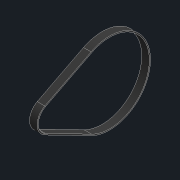
# Autodesk Inventor part: belt_1
Saved by Autodesk Inventor 2022 (Build 260153000, 153)
## iProperties
Created: 2021-07-18
Part Number: belt_1
Material: ゴム
Document SubType Name: Modeling
Designer: yuta0
Density: 0.93 g/cm^3
Appearance: ゴム - 黒
Mass: 8.55769 g
Surface Area: 248.449 cm^2
Volume: 9.20182 cm^3
購入先: ミスミ
在庫数: 0.0
Author: yuta0
Autodesk Inventor part; units mm, degrees
ref_plane "YZ Plane" through (0, 0, 0) normal (1, 0, 0) x (0, 1, 0)
ref_plane "XZ Plane" through (0, 0, 0) normal (0, 1, 0) x (-1, 0, 0)
ref_plane "XY Plane" through (0, 0, 0) normal (0, 0, 1) x (1, 0, 0)
sketch "スケッチ1" plane through (0, 0, 0) normal (1, 0, 0) x (0, 1, 0)
  arc A0 (15.5817, 7.9817) -> (-15.5817, 7.9817) centre (0, 0) ccw
  arc A1 (-46.7451, -52.855) -> (46.7451, -52.855) centre (0, -76.8) ccw
  line L0 (46.7451, -52.855) -> (15.5817, 7.9817)
  line L1 (-15.5817, 7.9817) -> (-46.7451, -52.855)
  arc A2 (16.4895, 8.4467) -> (-16.4895, 8.4467) centre (0, 0) ccw
  line L2 (-16.4895, 8.4467) -> (-47.6529, -52.3899)
  arc A3 (-47.6529, -52.3899) -> (47.6529, -52.3899) centre (0, -76.8) ccw
  line L3 (47.6529, -52.3899) -> (16.4895, 8.4467)
  arc A4 (15.1545, 7.7628) -> (-15.1545, 7.7628) centre (0, 0) ccw
  line L4 (-15.1545, 7.7628) -> (-46.3179, -53.0738)
  arc A5 (-46.3179, -53.0738) -> (46.3179, -53.0738) centre (0, -76.8) ccw
  line L5 (46.3179, -53.0738) -> (15.1545, 7.7628)
  dimension "d0" = 35.0141
  dimension "d1" = 105.0423
  dimension "d2" = 76.8
  dimension "d31" = 1.5
  dimension "d32" = 0.48
  constraints: 12 end point, 12 point on circle, 6 centre point, 5 tangent, 1 coincident, 1 vertical alignment, 4 other
  measures "d0" diameter of A0
  measures "d1" diameter of A1
  measures "d2" distance of A0.centre A1.centre
  measures "d31" distance between parallel lines of L3 L5
  measures "d32" distance between parallel lines of L5 L0
extrude "押し出し1" add sketch "スケッチ1" along normal mid plane 10 contours L0 A1 L1 A0 | L3 A3 L2 A2
